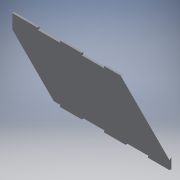
# Autodesk Inventor part: fechamento superior
Saved by Autodesk Inventor 2016 (Build 200138000, 138)
## iProperties
Created: 2017-06-07
Part Number: fechamento superior
Material: Generic
Document SubType Name: Modeling
Designer: fabio-note
Density: 1 g/cm^3
Appearance: Default
Author: fabio-note
Autodesk Inventor part; units mm, degrees
ref_plane "YZ Plane" through (0, 0, 0) normal (1, 0, 0) x (0, 1, 0)
ref_plane "XZ Plane" through (0, 0, 0) normal (0, 1, 0) x (-1, 0, 0)
ref_plane "XY Plane" through (0, 0, 0) normal (0, 0, 1) x (1, 0, 0)
sketch "Sketch1" plane through (0, 0, 0) normal (0, 1, 0) x (-1, 0, 0)
  line L0 (173, 61.75) -> (-173, 61.75)
  line L1 (-173, 61.75) -> (-173, -61.75)
  line L2 (-173, -61.75) -> (173, -61.75)
  line L3 (173, -61.75) -> (173, 61.75)
  point P0 (0, 0)
  point P1 (0, -61.75)
  point P2 (173, 0)
  dimension "d0" = 346
  dimension "d1" = 123.5
  constraints: 8 end point, 2 midpoint, 2 parallel, 1 horizontal, 1 horizontal alignment, 1 perpendicular, 1 vertical alignment
  measures "d0" distance between parallel lines of L3 L1
  measures "d1" distance between parallel lines of L0 L2
extrude "Extrusion1" add sketch "Sketch1" along normal blind 4
sketch "Esboço2" plane through (0, 4, 0) normal (0, 1, 0) x (1, 0, 0)
  line L0 (173, 61.75) -> (-173, 61.75) projected
  line L1 (118.5, 61.75) -> (70.5, 61.75)
  line L2 (70.5, 61.75) -> (70.5, 57.75)
  line L3 (70.5, 57.75) -> (118.5, 57.75)
  line L4 (118.5, 57.75) -> (118.5, 61.75)
  line L5 (173, -61.75) -> (173, 61.75) projected
  line L6 (24, 61.75) -> (-24, 61.75)
  line L7 (-24, 61.75) -> (-24, 57.75)
  line L8 (-24, 57.75) -> (24, 57.75)
  line L9 (24, 57.75) -> (24, 61.75)
  line L10 (-70.5, 61.75) -> (-118.5, 61.75)
  line L11 (-118.5, 61.75) -> (-118.5, 57.75)
  line L12 (-118.5, 57.75) -> (-70.5, 57.75)
  line L13 (-70.5, 57.75) -> (-70.5, 61.75)
  circle A0 centre (24, 57.75) radius 1
  circle A1 centre (70.5, 57.75) radius 1
  circle A2 centre (-24, 57.75) radius 1
  circle A3 centre (-70.5, 57.75) radius 1
  circle A4 centre (-118.5, 57.75) radius 1
  circle A5 centre (118.5, 57.75) radius 1
  point P0 (0, 0)
  dimension "d4" = 48
  dimension "d5" = 4
  dimension "d6" = 54.5
  dimension "d7" = 48
  dimension "d8" = 46.5
  dimension "d9" = 48
  dimension "d10" = 46.5
  dimension "d11" = 2
  dimension "d12" = 2
  dimension "d13" = 2
  dimension "d14" = 2
  dimension "d15" = 2
  dimension "d16" = 2
  constraints: 24 end point, 6 centre point, 6 coincident, 6 parallel, 3 horizontal, 3 perpendicular, 3 point on line
  measures "d4" distance of L3.end L2.end
  measures "d5" distance between parallel lines of L0 L3
  measures "d6" distance between parallel lines of L5 L4
  measures "d7" distance of L8.end L7.end
  measures "d8" distance between parallel lines of L9 L2
  measures "d9" distance of L12.end L11.end
  measures "d10" distance between parallel lines of L7 L13
  measures "d11" diameter of A0
  measures "d12" diameter of A1
  measures "d13" diameter of A2
  measures "d14" diameter of A3
  measures "d15" diameter of A4
  measures "d16" diameter of A5
extrude "Extrusão2" cut sketch "Esboço2" against normal blind 10
mirror "Espelhamento1" about plane through (0, 0, 0) normal (0, 0, 1) of "Extrusão2"
sketch "Esboço3" plane through (0, 4, 0) normal (0, 1, 0) x (1, 0, 0)
  line L0 (-118.5, 61.75) -> (-173, 61.75) projected
  line L1 (-173, 61.75) -> (-165, 61.75)
  line L2 (-165, 61.75) -> (-165, 21.75)
  line L3 (-165, 21.75) -> (-173, 21.75)
  line L4 (-173, 21.75) -> (-173, 61.75)
  line L5 (-173, 61.75) -> (-173, -61.75) projected
  line L6 (-173, -61.75) -> (-165, -61.75)
  line L7 (-165, -61.75) -> (-165, -21.75)
  line L8 (-165, -21.75) -> (-173, -21.75)
  line L9 (-173, -21.75) -> (-173, -61.75)
  circle A0 centre (-165, 21.75) radius 1
  circle A1 centre (-165, -21.75) radius 1
  point P0 (0, 0)
  dimension "d19" = 8
  dimension "d20" = 40
  dimension "d21" = 40
  dimension "d22" = 43.5
  dimension "d23" = 2
  dimension "d24" = 2
  constraints: 16 end point, 4 parallel, 2 centre point, 2 coincident, 2 horizontal, 2 perpendicular
  measures "d19" distance of L2.end L3.end
  measures "d20" distance between parallel lines of L0 L3
  measures "d21" distance between parallel lines of L8 L6
  measures "d22" distance between parallel lines of L3 L8
  measures "d23" diameter of A0
  measures "d24" diameter of A1
extrude "Extrusão3" cut sketch "Esboço3" against normal blind 10
mirror "Espelhamento2" about plane through (0, 0, 0) normal (1, 0, 0) of "Extrusão3"
body "Solid1"
